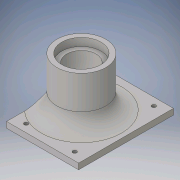
# Autodesk Inventor part: Tube
Saved by Autodesk Inventor 2016 (Build 200138000, 138)
## iProperties
Created: 2018-11-02
Part Number: Tube
Material: Generic
Document SubType Name: Modeling
Designer: attila
Density: 1 g/cm^3
Appearance: Default
Author: attila
Autodesk Inventor part; units mm, degrees
ref_plane "YZ Plane" through (0, 0, 0) normal (1, 0, 0) x (0, 1, 0)
ref_plane "XZ Plane" through (0, 0, 0) normal (0, 1, 0) x (-1, 0, 0)
ref_plane "XY Plane" through (0, 0, 0) normal (0, 0, 1) x (1, 0, 0)
sketch "Sketch1" plane through (0, 0, 0) normal (0, 1, 0) x (-1, 0, 0)
  line L0 (18.4, 24.2) -> (-18.4, 24.2)
  line L1 (-18.4, 24.2) -> (-18.4, -24.2)
  line L2 (-18.4, -24.2) -> (18.4, -24.2)
  line L3 (18.4, -24.2) -> (18.4, 24.2)
  point P0 (0, 0)
  point P1 (-18.4, 0)
  point P2 (0, -24.2)
  dimension "d0" = 48.4
  dimension "d1" = 36.8
  constraints: 8 end point, 2 midpoint, 2 parallel, 1 horizontal, 1 horizontal alignment, 1 perpendicular, 1 vertical alignment
  measures "d0" distance between parallel lines of L2 L0
  measures "d1" distance between parallel lines of L1 L3
extrude "Extrusion1" add sketch "Sketch1" along normal blind 3
sketch "Sketch2" plane through (0, 3, 0) normal (0, 1, 0) x (1, 0, 0)
  line L0 (-18.4, -24.2) -> (18.4, -24.2) projected
  line L1 (-18.4, 24.2) -> (-18.4, -24.2) projected
  line L2 (18.4, 24.2) -> (-18.4, 24.2) projected
  line L3 (18.4, -24.2) -> (18.4, 24.2) projected
  point P0 (0, 0)
  point P1 (-12.4, -20.2)
  point P2 (-12.4, 20.2)
  point P3 (12.4, -20.2)
  point P4 (12.4, 20.2)
  dimension "d4" = 4
  dimension "d5" = 6
  dimension "d6" = 6
  dimension "d7" = 4
  dimension "d8" = 6
  dimension "d9" = 4
  dimension "d10" = 6
  dimension "d11" = 4
  measures "d4" distance from line of L0 point (-12.4, -20.2)
  measures "d5" distance from line of L1 point (-12.4, 20.2)
  measures "d6" distance from line of L1 point (-12.4, -20.2)
  measures "d7" distance from line of L2 point (-12.4, 20.2)
  measures "d8" distance from line of L3 point (12.4, -20.2)
  measures "d9" distance from line of L0 point (12.4, -20.2)
  measures "d10" distance from line of L3 point (12.4, 20.2)
  measures "d11" distance from line of L2 point (12.4, 20.2)
hole "Hole1" at (-12.4, 3, 20.2) at (-12.4, 3, -20.2) at (12.4, 3, 20.2) at (12.4, 3, -20.2) direction (0, -1, 0) diameter 2 end through all
sketch "Sketch3" plane through (0, 3, 0) normal (0, 1, 0) x (1, 0, 0)
  line L0 (-18.4, 24.2) -> (-18.4, -24.2) projected
  line L1 (-18.4, -24.2) -> (18.4, -24.2) projected
  line L2 (18.4, 24.2) -> (-18.4, 24.2) projected
  circle A0 centre (-4.4, 0) radius 7.5
  circle A1 centre (-4.4, 0) radius 12.5
  point P0 (0, 0)
  dimension "d19" = 14
  dimension "d20" = 24.2
  dimension "d21" = 24.2
  dimension "d22" = 15
  dimension "d23" = 25
  constraints: 2 centre point, 2 coincident
  measures "d19" distance from line of L0 point (-4.4, 0)
  measures "d20" distance from line of L1 point (-4.4, 0)
  measures "d21" distance from line of L2 point (-4.4, 0)
  measures "d22" diameter of A0
  measures "d23" diameter of A1
extrude "Extrusion2" add sketch "Sketch3" along normal blind 25
sketch "Sketch4" plane through (-4.4, 3, 0) normal (0, 1, 0) x (1, 0, 0)
  circle A0 centre (0, 0) radius 7.5
  point P0 (4.4, 0)
  constraints: 1 centre point
extrude "Extrusion3" cut sketch "Sketch4" against normal blind 35
sketch "Sketch5" plane through (-4.4, 28, 0) normal (0, 1, 0) x (1, 0, 0)
  circle A0 centre (0, 0) radius 10
  point P0 (4.4, 0)
  dimension "d29" = 20
  constraints: 1 centre point
  measures "d29" diameter of A0
extrude "Extrusion4" cut sketch "Sketch5" against normal blind 4
sketch "Sketch8" plane through (0, 0, 0) normal (0, -1, 0) x (1, 0, 0)
  circle A0 centre (-4.4, 0) radius 7.5 projected
  circle A1 centre (-4.4, 0) radius 10
  point P0 (0, 0)
  dimension "d32" = 20
  constraints: 1 centre point, 1 coincident
  measures "d32" diameter of A1
extrude "Extrusion5" cut sketch "Sketch8" against normal blind 4
fillet "Fillet2" radius 8 1 edges at (-16.9, 3, 0)
equation "\"d20\" = d21"
body "Solid1"
